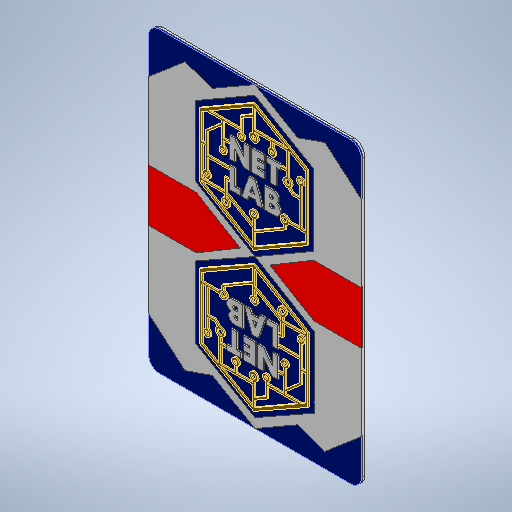
# Autodesk Inventor part: Aofwifi
Saved by Autodesk Inventor 2025 (Build 290162010, 162A)
## iProperties
Created: 2024-07-12
Part Number: Aofwifi
Material: Generic
Document SubType Name: Modeling
Designer: joshu
Density: 1 g/cm^3
Appearance: Default
Author: joshu
Autodesk Inventor part; units mm, degrees
(part 1 of 2)
ref_plane "YZ Plane" through (0, 0, 0) normal (1, 0, 0) x (0, 1, 0)
ref_plane "XZ Plane" through (0, 0, 0) normal (0, 1, 0) x (-1, 0, 0)
ref_plane "XY Plane" through (0, 0, 0) normal (0, 0, 1) x (1, 0, 0)
sketch "Sketch1" plane through (0, 0, 0) normal (0, 0, 1) x (1, 0, 0)
  line L0 (0, 0) -> (63.5, 0)
  line L1 (63.5, 0) -> (63.5, 88.9)
  line L2 (63.5, 88.9) -> (0, 88.9)
  line L3 (0, 88.9) -> (0, 0)
  line L4 (31.75, 44.45) -> (49.3079, 54.587)
  line L5 (49.3079, 54.587) -> (49.3079, 75.7826)
  line L6 (49.3079, 75.7826) -> (31.6801, 86.0828)
  line L7 (31.6801, 86.0828) -> (13.967, 75.8563)
  line L8 (13.967, 75.8563) -> (13.967, 55.04)
  line L9 (13.967, 55.04) -> (31.75, 44.45)
  line L10 (15.5263, 74.956) -> (31.6754, 84.2796)
  line L11 (31.6754, 84.2796) -> (47.7487, 74.8877)
  line L12 (47.7487, 74.8877) -> (47.7487, 55.4872)
  line L13 (47.7487, 55.4872) -> (31.7622, 46.2575)
  line L14 (31.7622, 46.2575) -> (15.5263, 55.9263)
  line L15 (15.5263, 55.9263) -> (15.5263, 74.956)
  line L16 (47.1273, 56.0392) -> (31.9379, 47.2671)
  line L17 (31.3664, 47.317) -> (16.2977, 56.192)
  line L18 (41.8086, 77.4972) -> (32.0418, 77.4972)
  line L19 (42.0908, 76.9257) -> (42.0908, 70.0939)
  line L20 (41.5193, 72.1376) -> (39.6994, 72.1376)
  line L21 (39.6994, 72.1376) -> (39.6994, 71.5661)
  line L22 (39.6994, 71.5661) -> (41.5193, 71.5661)
  arc A0 (31.465, 76.5861) -> (32.0365, 76.5861) centre (31.7507, 75.3324) ccw
  arc A1 (36.8763, 75.3571) -> (37.4478, 75.3571) centre (37.162, 74.2504) ccw
  circle A2 centre (37.162, 74.2504) radius 0.4762
  circle A3 centre (31.7507, 75.3324) radius 0.6191
  line L23 (45.9318, 69.8545) -> (45.9318, 58.9507)
  line L24 (45.3603, 66.7769) -> (43.3841, 66.7769)
  line L25 (43.1915, 66.2054) -> (45.3603, 66.2054)
  circle A4 centre (41.805, 68.7917) radius 0.762
  line L26 (43.1915, 66.2054) -> (41.9826, 67.4703)
  line L27 (43.3841, 66.7769) -> (42.5287, 67.6719)
  arc A5 (45.9318, 69.8545) -> (45.3603, 69.8545) centre (45.646, 70.9598) ccw
  circle A6 centre (45.646, 70.9598) radius 0.5715
  line L28 (40.6132, 56.5528) -> (40.6132, 57.4113)
  circle A7 centre (40.899, 58.665) radius 0.7144
  line L29 (32.0418, 83.1688) -> (32.0418, 77.4972)
  line L30 (32.0365, 76.9257) -> (32.0365, 76.5861)
  line L31 (32.0365, 76.9257) -> (36.8763, 76.9257)
  line L32 (36.8763, 75.3571) -> (36.8763, 76.9257)
  line L33 (37.4478, 76.9257) -> (37.4478, 75.3571)
  line L34 (37.4478, 76.9257) -> (41.5193, 76.9257)
  line L35 (42.0908, 76.9257) -> (42.7928, 76.9257)
  line L36 (32.0365, 83.1719) -> (41.8086, 77.4972)
  line L37 (42.7928, 76.9257) -> (47.1273, 74.4086)
  line L38 (41.5193, 70.0939) -> (41.5193, 71.5661)
  line L39 (41.5193, 72.1376) -> (41.5193, 76.9257)
  arc A8 (41.5193, 70.0939) -> (41.9826, 67.4703) centre (41.805, 68.7917) ccw
  arc A9 (42.5287, 67.6719) -> (42.0908, 70.0939) centre (41.805, 68.7917) ccw
  line L40 (45.3603, 58.9507) -> (45.3603, 66.2054)
  line L41 (45.3603, 66.7769) -> (45.3603, 69.8545)
  line L42 (47.1273, 58.9507) -> (45.9318, 58.9507)
  line L43 (45.3603, 58.9507) -> (42.1527, 58.9507)
  line L44 (42.1475, 58.3804) -> (47.1273, 58.3804)
  line L45 (41.1819, 57.4161) -> (41.1819, 56.2658)
  arc A10 (42.1527, 58.9507) -> (40.6132, 57.4113) centre (40.899, 58.665) ccw
  arc A11 (41.1819, 57.4161) -> (42.1475, 58.3804) centre (40.899, 58.665) ccw
  line L46 (47.1273, 74.4086) -> (47.1273, 58.9507)
  line L47 (47.1273, 58.3804) -> (47.1273, 56.0392)
  line L48 (27.6974, 78.6822) -> (27.6974, 79.0777)
  line L49 (28.2689, 78.6822) -> (31.465, 80.528)
  line L50 (27.6974, 79.0777) -> (31.465, 81.2535)
  line L51 (31.465, 76.5861) -> (31.465, 80.528)
  line L52 (31.465, 81.2535) -> (31.465, 83.1596)
  line L53 (31.9379, 51.4601) -> (40.6132, 56.5528)
  line L54 (31.9379, 50.8392) -> (41.1819, 56.2658)
  line L55 (16.2977, 57.1448) -> (22.9994, 57.1448)
  line L56 (22.9994, 56.5733) -> (16.2977, 56.5733)
  line L57 (16.2977, 56.5733) -> (16.2977, 57.1448)
  line L58 (22.9994, 60.9472) -> (23.5709, 60.9472)
  line L59 (22.9994, 60.9472) -> (24.4329, 60.9472)
  line L60 (24.4329, 60.9472) -> (24.4329, 60.3757)
  line L61 (24.4329, 60.3757) -> (23.5709, 60.3757)
  line L62 (22.9994, 60.3757) -> (22.9994, 60.9472)
  line L63 (23.5709, 56.4373) -> (31.3664, 51.9861)
  line L64 (31.3664, 52.5972) -> (23.5709, 57.0484)
  arc A12 (31.9379, 54.3552) -> (31.3664, 54.3552) centre (31.6521, 55.5111) ccw
  circle A13 centre (31.6521, 55.5111) radius 0.6191
  arc A14 (22.9994, 55.5805) -> (23.5709, 55.5805) centre (23.2852, 54.3309) ccw
  circle A15 centre (23.2852, 54.3309) radius 0.7144
  line L65 (23.5709, 60.3757) -> (23.5709, 57.0484)
  line L66 (23.5709, 56.4373) -> (23.5709, 55.5805)
  line L67 (22.9994, 55.5805) -> (22.9994, 56.5733)
  line L68 (22.9994, 57.1448) -> (22.9994, 60.9472)
  line L69 (31.3664, 54.3552) -> (31.3664, 52.5972)
  line L70 (31.3664, 51.9861) -> (31.3664, 47.317)
  line L71 (31.9379, 47.2671) -> (31.9379, 50.8392)
  line L72 (31.9379, 51.4601) -> (31.9379, 54.3552)
  arc A16 (27.6974, 74.6924) -> (28.2689, 74.6924) centre (27.9831, 73.6844) ccw
  circle A17 centre (27.9831, 73.6844) radius 0.4763
  line L73 (18.5492, 75.7007) -> (27.6974, 75.7007)
  line L74 (22.769, 70.6818) -> (24.4329, 70.6818)
  line L75 (24.4329, 70.6818) -> (24.4329, 70.1103)
  line L76 (24.4329, 70.1103) -> (22.769, 70.1103)
  line L77 (22.769, 70.1103) -> (22.769, 70.2009)
  line L78 (16.2977, 66.7769) -> (17.4065, 66.7769)
  line L79 (17.978, 66.7769) -> (17.978, 66.2054)
  line L80 (17.4065, 66.2054) -> (16.2977, 66.2054)
  line L81 (17.978, 63.9706) -> (24.4329, 63.9706)
  line L82 (24.4329, 63.9706) -> (24.4329, 63.3991)
  line L83 (24.4329, 63.3991) -> (17.978, 63.3991)
  line L84 (17.4065, 66.7769) -> (17.4065, 70.2549)
  line L85 (17.978, 70.0307) -> (17.978, 66.7769)
  line L86 (17.4065, 70.2549) -> (22.1975, 74.4365)
  line L87 (17.978, 70.0307) -> (22.1975, 73.7135)
  arc A18 (22.1975, 68.5281) -> (22.769, 68.5281) centre (22.4833, 67.4703) ccw
  circle A19 centre (22.4833, 67.4703) radius 0.5239
  line L88 (16.2977, 74.4004) -> (17.5596, 75.1292)
  line L89 (18.5492, 75.7007) -> (31.465, 83.1596)
  line L90 (27.6974, 75.1292) -> (22.769, 75.1292)
  line L91 (22.1975, 75.1292) -> (17.5596, 75.1292)
  line L92 (22.1975, 74.4365) -> (22.1975, 75.1292)
  line L93 (28.2689, 74.6924) -> (28.2689, 78.6822)
  line L94 (22.769, 75.1292) -> (22.769, 70.6818)
  line L95 (22.769, 70.1103) -> (22.769, 68.5281)
  line L96 (22.1975, 67.8875) -> (22.1975, 67.9094)
  line L97 (22.1975, 68.5281) -> (22.1975, 73.7135)
  line L98 (16.2977, 56.192) -> (16.2977, 66.2054)
  line L99 (16.2977, 66.7769) -> (16.2977, 74.4004)
  line L100 (17.978, 63.9706) -> (17.978, 66.2054)
  line L101 (27.6974, 78.6822) -> (27.6974, 75.7007)
  line L102 (27.6974, 75.1292) -> (27.6974, 74.6924)
  line L103 (24.4329, 66.1976) -> (26.1474, 66.1976)
  line L104 (26.1474, 66.1976) -> (26.1474, 69.7075)
  line L105 (26.1474, 72.4542) -> (24.4329, 72.4542)
  line L106 (24.4329, 72.4542) -> (24.4329, 66.1976)
  line L107 (28.7777, 72.4542) -> (30.4922, 72.4542)
  line L108 (30.4922, 72.4542) -> (30.4922, 66.1976)
  line L109 (30.4922, 66.1976) -> (28.7777, 66.1976)
  line L110 (28.7777, 68.9443) -> (28.7777, 72.4542)
  line L111 (28.7777, 66.1976) -> (26.1474, 69.7075)
  line L112 (26.1474, 72.4542) -> (28.7777, 68.9443)
  line L113 (31.2537, 72.4542) -> (32.9682, 72.4542)
  line L114 (32.9682, 66.1976) -> (31.2537, 66.1976)
  line L115 (31.2537, 66.1976) -> (31.2537, 72.4542)
  line L116 (31.2537, 72.4542) -> (34.8385, 72.4542)
  line L117 (34.8385, 72.4542) -> (34.8385, 70.7397)
  line L118 (34.8385, 70.7397) -> (32.9682, 70.7397)
  line L119 (31.2537, 70.7397) -> (31.2537, 72.4542)
  line L120 (32.9682, 70.0633) -> (34.8385, 70.0633)
  line L121 (34.8385, 70.0633) -> (34.8385, 68.5393)
  line L122 (34.8385, 68.5393) -> (32.9682, 68.5393)
  line L123 (31.2537, 68.5393) -> (31.2537, 70.0633)
  line L124 (31.2537, 66.1976) -> (34.8385, 66.1976)
  line L125 (34.8385, 66.1976) -> (34.8385, 67.9121)
  line L126 (34.8385, 67.9121) -> (32.9682, 67.9121)
  line L127 (31.2537, 67.9121) -> (31.2537, 66.1976)
  line L128 (32.9682, 70.7397) -> (32.9682, 70.0633)
  line L129 (32.9682, 68.5393) -> (32.9682, 67.9121)
  line L130 (39.6994, 72.4422) -> (35.4849, 72.4422)
  line L131 (35.4849, 72.4422) -> (35.4849, 70.9182)
  line L132 (39.6994, 70.9182) -> (39.6994, 72.4422)
  line L133 (38.4466, 70.9182) -> (38.4466, 66.1976)
  line L134 (38.4466, 66.1976) -> (36.7321, 66.1976)
  line L135 (36.7321, 66.1976) -> (36.7321, 70.9182)
  line L136 (36.7321, 70.9182) -> (36.8763, 70.9182)
  line L137 (35.4849, 70.9182) -> (36.7321, 70.9182)
  line L138 (38.4466, 70.9182) -> (39.6994, 70.9182)
  line L139 (24.4329, 64.6461) -> (26.1474, 64.6461)
  line L140 (26.1474, 64.6461) -> (26.1474, 59.9044)
  line L141 (26.1474, 58.3804) -> (24.4329, 58.3804)
  line L142 (24.4329, 58.3804) -> (24.4329, 64.6461)
  line L143 (24.4329, 58.3804) -> (27.8234, 58.3804)
  line L144 (27.8234, 58.3804) -> (27.8234, 59.9044)
  line L145 (27.8234, 59.9044) -> (26.1474, 59.9044)
  line L146 (24.4329, 59.9044) -> (24.4329, 58.3804)
  line L147 (28.1466, 58.3804) -> (29.8611, 58.3804)
  line L148 (29.8611, 58.3804) -> (30.3254, 59.5144)
  line L149 (30.3254, 59.5144) -> (32.2304, 59.5144)
  line L150 (30.3254, 64.6461) -> (32.2304, 64.6461)
  line L151 (28.1466, 58.3804) -> (30.3254, 64.6461)
  line L152 (32.728, 58.3804) -> (34.4425, 58.3804)
  line L153 (32.728, 58.3804) -> (32.2304, 59.5144)
  line L154 (34.4425, 58.3804) -> (32.2304, 64.6461)
  line L155 (30.6203, 60.8236) -> (31.9379, 60.8236)
  line L156 (31.9379, 60.8236) -> (31.2779, 62.4085)
  line L157 (31.2779, 62.4085) -> (30.6203, 60.8236)
  line L158 (34.9216, 58.3804) -> (34.9216, 64.6461)
  line L159 (34.9216, 64.6461) -> (37.8691, 64.6461)
  line L160 (34.9216, 58.3804) -> (37.8691, 58.3804)
  line L161 (36.5599, 59.8143) -> (36.5599, 60.939)
  line L162 (36.5599, 62.1736) -> (36.5599, 63.1944)
  line L163 (36.5599, 63.1944) -> (37.2133, 63.1944)
  line L164 (36.5599, 62.1736) -> (37.2133, 62.1736)
  arc A20 (37.2133, 62.1736) -> (37.2133, 63.1944) centre (37.055, 62.684) ccw
  line L165 (36.5599, 60.939) -> (37.4519, 60.939)
  line L166 (36.5599, 59.8143) -> (37.4396, 59.8143)
  arc A21 (37.4396, 59.8143) -> (37.4519, 60.939) centre (37.3959, 60.3772) ccw
  arc A22 (38.5631, 61.7817) -> (37.8691, 64.6461) centre (37.5266, 63.0469) ccw
  arc A23 (37.8691, 58.3804) -> (38.5631, 61.7817) centre (37.9604, 60.1332) ccw
  arc A24 (17.4065, 59.8724) -> (17.978, 59.8724) centre (17.6923, 58.815) ccw
  circle A25 centre (17.6923, 58.815) radius 0.5239
  line L167 (17.4065, 66.2054) -> (17.4065, 59.8724)
  line L168 (17.978, 59.8724) -> (17.978, 63.3991)
  line L169 (32.0418, 83.1688) -> (41.8086, 77.4972)
  line L170 (32.0418, 77.4972) -> (41.8086, 77.4972)
  line L171 (32.0418, 77.4972) -> (32.0418, 83.1688)
  line L172 (0, 44.45) -> (63.5, 44.45) construction
  line L173 (31.75, 88.9) -> (31.75, 0) construction
  line L174 (0, 52.2573) -> (14.2102, 52.2573)
  line L175 (14.2102, 52.2573) -> (27.3204, 44.45)
  line L176 (0, 36.6427) -> (14.2102, 36.6427)
  line L177 (14.2102, 36.6427) -> (27.3204, 44.45)
  line L178 (63.5, 52.2573) -> (49.2898, 52.2573)
  line L179 (49.2898, 52.2573) -> (36.1796, 44.45)
  line L180 (49.2898, 36.6427) -> (36.1796, 44.45)
  line L181 (63.5, 36.6427) -> (49.2898, 36.6427)
  line L182 (0, 75.0796) -> (10.8905, 84.3747)
  line L183 (10.8905, 84.3747) -> (18.9583, 81.5148)
  line L184 (18.9583, 81.5148) -> (31.75, 88.9)
  line L185 (63.5, 75.0796) -> (52.6095, 84.3747)
  line L186 (52.6095, 84.3747) -> (44.5417, 81.5148)
  line L187 (44.5417, 81.5148) -> (31.75, 88.9)
  line L188 (46.0393, 22.6946) -> (47.1481, 22.6946)
  line L189 (45.4678, 22.1231) -> (45.4678, 22.6946)
  line L190 (45.4678, 24.9294) -> (45.4678, 22.6946)
  line L191 (47.1481, 22.1231) -> (46.0393, 22.1231)
  line L192 (47.1481, 32.3267) -> (47.1481, 31.7552)
  line L193 (47.1481, 32.708) -> (47.1481, 22.6946)
  line L194 (47.1481, 31.7552) -> (40.4464, 31.7552)
  line L195 (40.4464, 32.3267) -> (47.1481, 32.3267)
  line L196 (45.4678, 29.0276) -> (45.4678, 25.5009)
  line L197 (46.0393, 22.6946) -> (46.0393, 29.0276)
  circle A26 centre (45.7535, 30.085) radius 0.5239
  arc A27 (46.0393, 29.0276) -> (45.4678, 29.0276) centre (45.7535, 30.085) ccw
  line L198 (20.6531, 11.9743) -> (16.3185, 14.4914)
  line L199 (21.355, 11.9743) -> (20.6531, 11.9743)
  line L200 (21.9265, 16.7624) -> (21.9265, 11.9743)
  line L201 (21.355, 11.9743) -> (21.355, 18.8061)
  line L202 (21.9265, 16.7624) -> (23.7464, 16.7624)
  line L203 (23.7464, 17.3339) -> (21.9265, 17.3339)
  line L204 (25.998, 11.9743) -> (21.9265, 11.9743)
  line L205 (26.5695, 13.5429) -> (26.5695, 11.9743)
  circle A28 centre (21.6408, 20.1083) radius 0.762
  circle A29 centre (26.2838, 14.6496) radius 0.4762
  arc A30 (26.5695, 13.5429) -> (25.998, 13.5429) centre (26.2838, 14.6496) ccw
  line L206 (31.4093, 11.9743) -> (26.5695, 11.9743)
  arc A31 (31.9808, 12.3139) -> (31.4093, 12.3139) centre (31.6951, 13.5676) ccw
  line L207 (25.998, 11.9743) -> (25.998, 13.5429)
  line L208 (45.4678, 24.9294) -> (39.013, 24.9294)
  line L209 (39.013, 25.5009) -> (45.4678, 25.5009)
  line L210 (39.013, 24.9294) -> (39.013, 25.5009)
  circle A32 centre (40.1606, 34.5691) radius 0.7144
  arc A33 (40.4464, 33.3195) -> (39.8749, 33.3195) centre (40.1606, 34.5691) ccw
  line L211 (39.8749, 32.4627) -> (39.8749, 33.3195)
  line L212 (40.4464, 33.3195) -> (40.4464, 32.3267)
  line L213 (39.013, 27.9528) -> (39.013, 28.5243)
  line L214 (39.8749, 28.5243) -> (39.8749, 31.8516)
  line L215 (39.013, 28.5243) -> (39.8749, 28.5243)
  line L216 (40.4464, 31.7552) -> (40.4464, 27.9528)
  line L217 (40.4464, 28.5243) -> (40.4464, 27.9528)
  line L218 (40.4464, 27.9528) -> (39.8749, 27.9528)
  line L219 (40.4464, 27.9528) -> (39.013, 27.9528)
  line L220 (33.5847, 30.5196) -> (33.1204, 29.3856)
  line L221 (35.6224, 28.9956) -> (37.2985, 28.9956)
  line L222 (35.2992, 30.5196) -> (33.5847, 30.5196)
  line L223 (39.013, 28.9956) -> (39.013, 30.5196)
  line L224 (35.2992, 30.5196) -> (33.1204, 24.2539)
  line L225 (46.0393, 18.6451) -> (41.2483, 14.4635)
  line L226 (45.4678, 18.8693) -> (41.2483, 15.1865)
  line L227 (40.6768, 18.7897) -> (40.6768, 20.3719)
  line L228 (41.2483, 21.0125) -> (41.2483, 20.9906)
  line L229 (41.2483, 20.3719) -> (41.2483, 15.1865)
  line L230 (40.6768, 13.7708) -> (40.6768, 18.2182)
  line L231 (41.2483, 14.4635) -> (41.2483, 13.7708)
  line L232 (41.2483, 13.7708) -> (45.8862, 13.7708)
  line L233 (47.1481, 22.1231) -> (47.1481, 14.4996)
  line L234 (47.1481, 14.4996) -> (45.8862, 13.7708)
  circle A34 centre (40.9626, 21.4297) radius 0.5239
  line L235 (32.8255, 28.0764) -> (31.5079, 28.0764)
  line L236 (32.1679, 26.4915) -> (32.8255, 28.0764)
  line L237 (31.5079, 28.0764) -> (32.1679, 26.4915)
  line L238 (33.1204, 29.3856) -> (31.2154, 29.3856)
  line L239 (35.6224, 30.5196) -> (35.6224, 28.9956)
  line L240 (37.2985, 24.2539) -> (37.2985, 28.9956)
  line L241 (37.2985, 30.5196) -> (39.013, 30.5196)
  line L242 (39.013, 30.5196) -> (39.013, 24.2539)
  line L243 (39.013, 30.5196) -> (35.6224, 30.5196)
  line L244 (39.013, 24.2539) -> (37.2985, 24.2539)
  line L245 (33.1204, 24.2539) -> (31.2154, 24.2539)
  line L246 (30.7178, 30.5196) -> (31.2154, 29.3856)
  line L247 (37.2985, 16.4458) -> (39.013, 16.4458)
  line L248 (40.6768, 18.2182) -> (39.013, 18.2182)
  line L249 (39.013, 18.7897) -> (40.6768, 18.7897)
  line L250 (40.6768, 18.7897) -> (40.6768, 18.6991)
  line L251 (39.013, 18.2182) -> (39.013, 18.7897)
  line L252 (46.0393, 22.1231) -> (46.0393, 18.6451)
  line L253 (45.4678, 18.8693) -> (45.4678, 22.1231)
  arc A35 (41.2483, 20.3719) -> (40.6768, 20.3719) centre (40.9626, 21.4297) ccw
  line L254 (39.013, 16.4458) -> (39.013, 22.7024)
  line L255 (39.013, 22.7024) -> (37.2985, 22.7024)
  line L256 (32.9536, 22.7024) -> (34.6681, 22.7024)
  line L257 (30.4777, 22.7024) -> (32.1922, 22.7024)
  line L258 (30.4777, 18.8367) -> (28.6073, 18.8367)
  line L259 (32.1922, 22.7024) -> (28.6073, 22.7024)
  line L260 (28.6073, 22.7024) -> (28.6073, 20.9879)
  line L261 (28.6073, 20.9879) -> (30.4777, 20.9879)
  line L262 (32.1922, 20.9879) -> (32.1922, 22.7024)
  line L263 (30.4777, 20.3607) -> (30.4777, 20.9879)
  line L264 (28.6073, 20.3607) -> (30.4777, 20.3607)
  line L265 (28.6073, 18.8367) -> (28.6073, 20.3607)
  line L266 (32.1922, 20.3607) -> (32.1922, 18.8367)
  line L267 (30.4777, 18.1603) -> (30.4777, 18.8367)
  line L268 (26.8859, 25.7056) -> (26.2325, 25.7056)
  line L269 (26.8859, 29.0857) -> (26.0062, 29.0857)
  line L270 (26.8859, 27.961) -> (25.9939, 27.961)
  line L271 (28.5242, 30.5196) -> (25.5767, 30.5196)
  line L272 (32.0794, 36.9139) -> (32.0794, 41.583)
  line L273 (31.5079, 41.6329) -> (31.5079, 38.0608)
  line L274 (26.8859, 26.7264) -> (26.8859, 25.7056)
  line L275 (28.5242, 24.2539) -> (25.5767, 24.2539)
  line L276 (29.0033, 30.5196) -> (31.2154, 24.2539)
  line L277 (30.7178, 30.5196) -> (29.0033, 30.5196)
  line L278 (26.8859, 26.7264) -> (26.2325, 26.7264)
  line L279 (28.5242, 30.5196) -> (28.5242, 24.2539)
  arc A36 (26.2325, 26.7264) -> (26.2325, 25.7056) centre (26.3908, 26.216) ccw
  line L280 (26.8859, 29.0857) -> (26.8859, 27.961)
  arc A37 (26.0062, 29.0857) -> (25.9939, 27.961) centre (26.0499, 28.5228) ccw
  arc A38 (24.8827, 27.1183) -> (25.5767, 24.2539) centre (25.9192, 25.8531) ccw
  arc A39 (25.5767, 30.5196) -> (24.8827, 27.1183) centre (25.4854, 28.7668) ccw
  line L281 (23.7464, 16.7624) -> (23.7464, 17.3339)
  line L282 (24.9992, 22.7024) -> (26.7137, 22.7024)
  line L283 (27.961, 17.9818) -> (26.7137, 17.9818)
  line L284 (26.7137, 22.7024) -> (26.7137, 17.9818)
  line L285 (26.7137, 17.9818) -> (26.5695, 17.9818)
  line L286 (24.9992, 17.9818) -> (24.9992, 22.7024)
  line L287 (24.9992, 17.9818) -> (23.7464, 17.9818)
  line L288 (27.961, 16.4578) -> (27.961, 17.9818)
  line L289 (23.7464, 16.4578) -> (27.961, 16.4578)
  line L290 (23.7464, 17.9818) -> (23.7464, 16.4578)
  line L291 (31.75, 44.45) -> (14.1379, 34.5158)
  line L292 (15.6972, 33.6051) -> (31.7276, 42.6471)
  line L293 (16.3185, 32.8608) -> (31.5079, 41.6329)
  line L294 (31.5079, 37.4399) -> (22.8326, 32.3472)
  line L295 (31.5079, 38.0608) -> (22.2639, 32.6342)
  line L296 (31.5079, 37.4399) -> (31.5079, 34.5448)
  line L297 (35.7484, 10.2178) -> (35.7484, 9.8223)
  line L298 (35.1769, 10.2178) -> (31.9808, 8.372)
  line L299 (35.7484, 9.8223) -> (31.9808, 7.6465)
  line L300 (31.9808, 12.3139) -> (31.9808, 8.372)
  line L301 (31.9808, 7.6465) -> (31.9808, 5.7404)
  circle A40 centre (35.4627, 15.2156) radius 0.4763
  arc A41 (35.7484, 14.2076) -> (35.1769, 14.2076) centre (35.4627, 15.2156) ccw
  line L302 (35.7484, 13.7708) -> (35.7484, 14.2076)
  line L303 (35.7484, 13.7708) -> (40.6768, 13.7708)
  line L304 (44.8966, 13.1993) -> (35.7484, 13.1993)
  line L305 (35.1769, 14.2076) -> (35.1769, 10.2178)
  line L306 (35.7484, 10.2178) -> (35.7484, 13.1993)
  line L307 (44.8966, 13.1993) -> (31.9808, 5.7404)
  line L308 (31.4093, 11.9743) -> (31.4093, 12.3139)
  line L309 (47.9195, 13.7706) -> (31.7623, 4.657)
  circle A42 centre (31.6951, 13.5676) radius 0.6191
  line L310 (31.7499, 2.8598) -> (49.4788, 12.8599)
  line L311 (47.9195, 32.9751) -> (47.9195, 13.7706)
  line L312 (49.4788, 12.8599) -> (49.4788, 33.86)
  circle A43 centre (31.7937, 33.3889) radius 0.6191
  line L313 (32.0794, 41.583) -> (47.1481, 32.708)
  line L314 (49.4788, 33.86) -> (31.75, 44.45)
  line L315 (31.7276, 42.6471) -> (47.9195, 32.9751)
  line L316 (32.0794, 36.3028) -> (39.8749, 31.8516)
  line L317 (39.8749, 32.4627) -> (32.0794, 36.9139)
  line L318 (32.0794, 34.5448) -> (32.0794, 36.3028)
  arc A44 (31.5079, 34.5448) -> (32.0794, 34.5448) centre (31.7937, 33.3889) ccw
  circle A45 centre (17.7998, 17.9402) radius 0.5715
  line L319 (18.0855, 22.1231) -> (20.0617, 22.1231)
  line L320 (20.2543, 22.6946) -> (18.0855, 22.6946)
  line L321 (22.8326, 32.3472) -> (22.8326, 31.4887)
  circle A46 centre (22.5468, 30.235) radius 0.7144
  line L322 (21.2984, 30.5196) -> (16.3185, 30.5196)
  line L323 (22.2639, 31.4839) -> (22.2639, 32.6342)
  arc A47 (21.2931, 29.9493) -> (22.8326, 31.4887) centre (22.5468, 30.235) ccw
  arc A48 (22.2639, 31.4839) -> (21.2984, 30.5196) centre (22.5468, 30.235) ccw
  line L324 (16.3185, 30.5196) -> (16.3185, 32.8608)
  line L325 (14.1379, 34.5158) -> (14.1379, 13.1174)
  line L326 (15.6972, 14.0137) -> (15.6972, 33.6051)
  line L327 (17.514, 19.0455) -> (17.514, 29.9493)
  line L328 (20.2543, 22.6946) -> (21.4633, 21.4297)
  line L329 (20.0617, 22.1231) -> (20.9171, 21.2281)
  arc A49 (17.514, 19.0455) -> (18.0855, 19.0455) centre (17.7998, 17.9402) ccw
  line L330 (21.9265, 18.8061) -> (21.9265, 17.3339)
  arc A50 (20.9171, 21.2281) -> (21.355, 18.8061) centre (21.6408, 20.1083) ccw
  line L331 (18.0855, 22.1231) -> (18.0855, 19.0455)
  line L332 (16.3185, 14.4914) -> (16.3185, 29.9493)
  line L333 (16.3185, 29.9493) -> (17.514, 29.9493)
  line L334 (18.0855, 29.9493) -> (18.0855, 22.6946)
  line L335 (18.0855, 29.9493) -> (21.2931, 29.9493)
  arc A51 (21.9265, 18.8061) -> (21.4633, 21.4297) centre (21.6408, 20.1083) ccw
  line L336 (14.1379, 13.1174) -> (31.7499, 2.8598)
  line L337 (31.7623, 4.657) -> (15.6972, 14.0137)
  line L338 (21.6372, 11.4028) -> (31.404, 11.4028)
  line L339 (31.404, 11.4028) -> (31.404, 5.7312)
  line L340 (31.404, 5.7312) -> (21.6372, 11.4028)
  line L341 (37.2985, 22.7024) -> (37.2985, 19.1925)
  line L342 (34.6681, 16.4458) -> (32.9536, 16.4458)
  line L343 (32.9536, 16.4458) -> (32.9536, 22.7024)
  line L344 (34.6681, 22.7024) -> (37.2985, 19.1925)
  line L345 (28.6073, 18.1603) -> (30.4777, 18.1603)
  line L346 (32.1922, 16.4458) -> (28.6073, 16.4458)
  line L347 (28.6073, 16.4458) -> (28.6073, 18.1603)
  line L348 (32.1922, 22.7024) -> (32.1922, 16.4458)
  line L349 (32.1922, 16.4458) -> (30.4777, 16.4458)
  line L350 (34.6681, 19.9557) -> (34.6681, 16.4458)
  line L351 (37.2985, 16.4458) -> (34.6681, 19.9557)
  line L352 (32.1922, 18.1603) -> (32.1922, 16.4458)
  line L353 (0, 13.8204) -> (10.8905, 4.5253)
  line L354 (10.8905, 4.5253) -> (18.9583, 7.3852)
  line L355 (18.9583, 7.3852) -> (31.75, 0)
  line L356 (63.5, 13.8204) -> (52.6095, 4.5253)
  line L357 (52.6095, 4.5253) -> (44.5417, 7.3852)
  line L358 (44.5417, 7.3852) -> (31.75, 0)
  point P0 (31.9379, 47.317)
  point P1 (31.7229, 65.2666)
  point P2 (31.7229, 23.6334)
  point P3 (31.7229, 23.6334)
  point P4 (31.9379, 5.6837)
  point P5 (63.5, 75.0796)
  dimension "d0" = 63.5
  dimension "d1" = 88.9
  dimension "d43" = 44.45
  dimension "d99" = 120
  constraints: 718 end point, 170 parallel, 64 point on circle, 50 centre point, 42 perpendicular, 36 horizontal, 21 point on line, 20 coincident, 19 symmetric about line, 7 collinear, 5 midpoint, 4 vertical, 17 other
  measures "d0" distance of L2.end L1.end
  measures "d1" distance of L1.end L0.end
  measures "d43" distance between parallel lines of L172 L2
  measures "d99" angle of L357 L356
extrude "Extrusion1" add sketch "Sketch1" along normal blind 0.4 contours L3 L353 L354 L355 L0 | L358 L357 L356 L1 L0 | L3 L2 L184 L183 L182 | L185 L186 L187 L2 L1 | L9 L8 L7 L6 L5 L4 | L314 L312 L310 L336 L325 L291 | L10 L11 L12 L13 L14 L15 | L16 L71 L54 L45 A11 L44 L47 | L17 L98 L56 L67 A14 L66 L63 L70 | L18 L29 L36 | L35 L37 L46 L42 L23 A5 L41 L24 L27 A9 L19 | L20 L132 L130 L131 L137 L135 L134 L133 L138 L22 L38 A8 L26 L25 L40 L43 A10 L28 L53 L72 A12 L69 L64 L65 L61 L142 L141 L143 L144 L145 L140 L139 L81 L100 L79 L85 L87 L97 A18 L95 L76 L106 L103 L104 L111 L109 L108 L107 L110 L112 L105 L74 L94 L90 L102 A16 L93 L49 L51 A0 L30 L31 L32 A1 L33 L34 L39 | L21 L132 L138 L133 L134 L135 L137 L131 L130 | L106 L105 L112 L110 L107 L108 L109 L111 L104 L103 L75 | L60 L142 L82 L139 L140 L145 L144 L143 L141 | L59 L58 L62 L68 L55 L98 L80 L167 A24 L168 L83 L142 | A2 | A3 | A4 | A6 | A7 | L101 L73 L89 L52 L50 L48 | A13 | A15 | A17 | L99 L88 L91 L92 L86 L84 L78 | A19 | L113 L116 L117 L118 L128 L120 L121 L122 L129 L126 L125 L124 L114 L115 | L151 L150 L154 L152 L153 L149 L148 L147 | L157 L156 L155 | L158 L159 A22 A23 L160 | L161 L165 A21 L166 | L162 L163 A20 L164 | A25 | L197 A27 L196 L209 L242 L219 L218 L216 L194 L193 L188 | L210 L242 L244 L240 L221 L239 L243 L241 L223 L213 | L208 L190 L189 L253 L226 L229 A35 L227 L249 L254 L255 L341 L344 L256 L343 L342 L350 L351 L247 L248 L230 L303 L302 A41 L305 L298 L300 A31 L308 L206 L205 A30 L207 L204 L200 L202 L290 L289 L288 L283 L284 L282 L286 L287 L203 L330 A51 L328 L320 L334 L335 A47 L321 L294 L296 A44 L318 L316 L214 L215 L242 L223 L241 L243 L239 L221 L240 L244 | L251 L254 L247 L351 L350 L342 L343 L256 L344 L341 L255 | L290 L287 L286 L282 L284 L283 L288 L289 L281 | L233 L234 L232 L231 L225 L252 L191 | L193 L195 L212 A33 L211 L317 L272 L313 | A26 | L198 L332 L333 L327 A49 L331 L319 L329 A50 L201 L199 | A28 | A29 | A32 | L222 L224 L245 L276 L277 L246 L238 L220 | A34 | L236 L237 L235 | L257 L262 L348 L266 L346 L347 L345 L267 L258 L265 L264 L263 L261 L260 L259 | L268 A36 L278 L274 | L280 L270 A37 L269 | L279 L275 A38 A39 L271 | L273 L295 L323 A48 L322 L324 L293 | L292 L315 L311 L309 L337 L326 | L306 L304 L307 L301 L299 L297 | A40 | A42 | A43 | A45 | A46 | L338 L339 L340
extrude "Extrusion12" add sketch "Sketch1" along normal blind 0.4 separate body contours L3 L174 L175 L177 L176 | L181 L180 L179 L178 L1
extrude "Extrusion13" add sketch "Sketch1" along normal blind 0.4 separate body contours L355 L354 L353 L3 L176 L177 L175 L174 L182 L183 L184 L187 L186 L185 L1 L178 L179 L180 L181 L356 L357 L358
extrude "Extrusion14" add sketch "Sketch1" against normal blind 0.4 contours L21 L132 L138 L133 L134 L135 L137 L131 L130 | L106 L105 L112 L110 L107 L108 L109 L111 L104 L103 L75 | L60 L142 L82 L139 L140 L145 L144 L143 L141 | L113 L116 L117 L118 L128 L120 L121 L122 L129 L126 L125 L124 L114 L115 | L151 L150 L154 L152 L153 L149 L148 L147 | L158 L159 A22 A23 L160 | L210 L242 L244 L240 L221 L239 L243 L241 L223 L213 | L251 L254 L247 L351 L350 L342 L343 L256 L344 L341 L255 | L290 L287 L286 L282 L284 L283 L288 L289 L281 | L222 L224 L245 L276 L277 L246 L238 L220 | L257 L262 L348 L266 L346 L347 L345 L267 L258 L265 L264 L263 L261 L260 L259 | L279 L275 A38 A39 L271 bodies 3
extrude "Extrusion15" add sketch "Sketch1" against normal blind 0.4 separate body contours L10 L11 L12 L13 L14 L15 | L292 L315 L311 L309 L337 L326
pattern_linear "Rectangular Pattern1" count 2 spacing 0.8 along (0, 0, 1) of "Extrusion15" bodies 4
pattern_linear "Rectangular Pattern2" count 2 spacing 0.8 along (0, 0, 1) of "Extrusion14" bodies 3
extrude "Extrusion16" cut sketch "Sketch1" against normal blind 0.4 contours L9 L8 L7 L6 L5 L4 | L314 L312 L310 L336 L325 L291 | L10 L11 L12 L13 L14 L15 | L16 L71 L54 L45 A11 L44 L47 | L17 L98 L56 L67 A14 L66 L63 L70 | L18 L29 L36 | L35 L37 L46 L42 L23 A5 L41 L24 L27 A9 L19 | L20 L132 L130 L131 L137 L135 L134 L133 L138 L22 L38 A8 L26 L25 L40 L43 A10 L28 L53 L72 A12 L69 L64 L65 L61 L142 L141 L143 L144 L145 L140 L139 L81 L100 L79 L85 L87 L97 A18 L95 L76 L106 L103 L104 L111 L109 L108 L107 L110 L112 L105 L74 L94 L90 L102 A16 L93 L49 L51 A0 L30 L31 L32 A1 L33 L34 L39 | L21 L132 L138 L133 L134 L135 L137 L131 L130 | L106 L105 L112 L110 L107 L108 L109 L111 L104 L103 L75 | L60 L142 L82 L139 L140 L145 L144 L143 L141 | L59 L58 L62 L68 L55 L98 L80 L167 A24 L168 L83 L142 | A2 | A3 | A4 | A6 | A7 | L101 L73 L89 L52 L50 L48 | A13 | A15 | A17 | L99 L88 L91 L92 L86 L84 L78 | A19 | L113 L116 L117 L118 L128 L120 L121 L122 L129 L126 L125 L124 L114 L115 | L151 L150 L154 L152 L153 L149 L148 L147 | L157 L156 L155 | L158 L159 A22 A23 L160 | L161 L165 A21 L166 | L162 L163 A20 L164 | A25 | L197 A27 L196 L209 L242 L219 L218 L216 L194 L193 L188 | L210 L242 L244 L240 L221 L239 L243 L241 L223 L213 | L208 L190 L189 L253 L226 L229 A35 L227 L249 L254 L255 L341 L344 L256 L343 L342 L350 L351 L247 L248 L230 L303 L302 A41 L305 L298 L300 A31 L308 L206 L205 A30 L207 L204 L200 L202 L290 L289 L288 L283 L284 L282 L286 L287 L203 L330 A51 L328 L320 L334 L335 A47 L321 L294 L296 A44 L318 L316 L214 L215 L242 L223 L241 L243 L239 L221 L240 L244 | L251 L254 L247 L351 L350 L342 L343 L256 L344 L341 L255 | L290 L287 L286 L282 L284 L283 L288 L289 L281 | L233 L234 L232 L231 L225 L252 L191 | L193 L195 L212 A33 L211 L317 L272 L313 | A26 | L198 L332 L333 L327 A49 L331 L319 L329 A50 L201 L199 | A28 | A29 | A32 | L222 L224 L245 L276 L277 L246 L238 L220 | A34 | L236 L237 L235 | L257 L262 L348 L266 L346 L347 L345 L267 L258 L265 L264 L263 L261 L260 L259 | L268 A36 L278 L274 | L280 L270 A37 L269 | L279 L275 A38 A39 L271 | L273 L295 L323 A48 L322 L324 L293 | L292 L315 L311 L309 L337 L326 | L306 L304 L307 L301 L299 L297 | A40 | A42 | A43 | A45 | A46 | L338 L339 L340 bodies 3
extrude "Extrusion17" cut sketch "Sketch1" against normal blind 25.4 contours L9 L8 L7 L6 L5 L4 | L314 L312 L310 L336 L325 L291 | L10 L11 L12 L13 L14 L15 | L16 L71 L54 L45 A11 L44 L47 | L17 L98 L56 L67 A14 L66 L63 L70 | L18 L29 L36 | L35 L37 L46 L42 L23 A5 L41 L24 L27 A9 L19 | L20 L132 L130 L131 L137 L135 L134 L133 L138 L22 L38 A8 L26 L25 L40 L43 A10 L28 L53 L72 A12 L69 L64 L65 L61 L142 L141 L143 L144 L145 L140 L139 L81 L100 L79 L85 L87 L97 A18 L95 L76 L106 L103 L104 L111 L109 L108 L107 L110 L112 L105 L74 L94 L90 L102 A16 L93 L49 L51 A0 L30 L31 L32 A1 L33 L34 L39 | L21 L132 L138 L133 L134 L135 L137 L131 L130 | L106 L105 L112 L110 L107 L108 L109 L111 L104 L103 L75 | L60 L142 L82 L139 L140 L145 L144 L143 L141 | L59 L58 L62 L68 L55 L98 L80 L167 A24 L168 L83 L142 | A2 | A3 | A4 | A6 | A7 | L101 L73 L89 L52 L50 L48 | A13 | A15 | A17 | L99 L88 L91 L92 L86 L84 L78 | A19 | L113 L116 L117 L118 L128 L120 L121 L122 L129 L126 L125 L124 L114 L115 | L151 L150 L154 L152 L153 L149 L148 L147 | L157 L156 L155 | L158 L159 A22 A23 L160 | L161 L165 A21 L166 | L162 L163 A20 L164 | A25 | L197 A27 L196 L209 L242 L219 L218 L216 L194 L193 L188 | L210 L242 L244 L240 L221 L239 L243 L241 L223 L213 | L208 L190 L189 L253 L226 L229 A35 L227 L249 L254 L255 L341 L344 L256 L343 L342 L350 L351 L247 L248 L230 L303 L302 A41 L305 L298 L300 A31 L308 L206 L205 A30 L207 L204 L200 L202 L290 L289 L288 L283 L284 L282 L286 L287 L203 L330 A51 L328 L320 L334 L335 A47 L321 L294 L296 A44 L318 L316 L214 L215 L242 L223 L241 L243 L239 L221 L240 L244 | L251 L254 L247 L351 L350 L342 L343 L256 L344 L341 L255 | L290 L287 L286 L282 L284 L283 L288 L289 L281 | L233 L234 L232 L231 L225 L252 L191 | L193 L195 L212 A33 L211 L317 L272 L313 | A26 | L198 L332 L333 L327 A49 L331 L319 L329 A50 L201 L199 | A28 | A29 | A32 | L222 L224 L245 L276 L277 L246 L238 L220 | A34 | L236 L237 L235 | L257 L262 L348 L266 L346 L347 L345 L267 L258 L265 L264 L263 L261 L260 L259 | L268 A36 L278 L274 | L280 L270 A37 L269 | L279 L275 A38 A39 L271 | L273 L295 L323 A48 L322 L324 L293 | L292 L315 L311 L309 L337 L326 | L306 L304 L307 L301 L299 L297 | A40 | A42 | A43 | A45 | A46 | L338 L339 L340 bodies 4
sketch "Sketch14" plane through (0, 0, 0) normal (0, 0, -1) x (-1, 0, 0)
  line L0 (-63.5, 75.0796) -> (-63.5, 88.9) projected
  line L1 (0, 0) -> (-63.5, 0)
  line L2 (-63.5, 0) -> (-63.5, 88.9)
  line L3 (-63.5, 88.9) -> (0, 88.9)
  line L4 (0, 88.9) -> (0, 0)
  line L5 (-62.5, 1) -> (-1, 1)
  line L6 (-1, 1) -> (-1, 87.9)
  line L7 (-1, 87.9) -> (-62.5, 87.9)
  line L8 (-62.5, 87.9) -> (-62.5, 1)
  dimension "d90" = 1
  constraints: 16 end point, 4 parallel, 2 perpendicular, 1 horizontal, 3 other
  measures "d90" distance between parallel lines of L1 L5
extrude "Extrusion18" add sketch "Sketch14" along normal blind 0.2 separate body contours L8 L7 L6 L5
sketch "Sketch16" plane through (0, 0, 0) normal (0, 0, -1) x (-1, 0, 0)
  line L0 (-1, 1) -> (-1, 87.9) projected
  line L1 (-1, 87.9) -> (-62.5, 87.9) projected
  line L2 (-62.5, 87.9) -> (-62.5, 1) projected
  line L3 (-62.5, 1) -> (-1, 1) projected
  line L4 (0, 88.9) -> (0, 75.0796) projected
  line L5 (-31.75, 0) -> (-63.5, 0) projected
  line L6 (0, 88.9) -> (-63.5, 88.9)
  line L7 (-63.5, 88.9) -> (-63.5, 0)
  line L8 (-63.5, 0) -> (0, 0)
  line L9 (0, 0) -> (0, 88.9)
  constraints: 8 end point, 2 parallel, 1 horizontal, 1 perpendicular
extrude "Extrusion19" add sketch "Sketch16" along normal blind 0.2 bodies 3
sketch "Sketch17" plane through (0, 0, -0.2) normal (0, 0, -1) x (-1, 0, 0)
  line L0 (-63.5, 88.9) -> (-63.5, 0)
  line L1 (-63.5, 0) -> (0, 0)
  line L2 (0, 0) -> (0, 88.9)
  line L3 (0, 88.9) -> (-63.5, 88.9)
  line L4 (-62.5, 1) -> (-62.5, 87.9) construction
  line L5 (-62.5, 44.45) -> (-1, 44.45) construction
  line L6 (-1, 87.9) -> (-1, 1) construction
  line L7 (-57.9556, 87.392) -> (-49.5403, 87.392) construction
  line L8 (-49.5403, 87.392) -> (-49.5403, 73.7102) construction
  line L9 (-49.5403, 73.7102) -> (-57.9556, 73.7102) construction
  line L10 (-57.9556, 73.7102) -> (-57.9556, 87.392) construction
  line L11 (-5.5444, 1.508) -> (-13.9597, 1.508) construction
  line L12 (-13.9597, 1.508) -> (-13.9597, 15.8789) construction
  line L13 (-13.9597, 15.8789) -> (-5.5444, 15.8789) construction
  line L14 (-5.5444, 15.8789) -> (-5.5444, 1.508) construction
  line L15 (-62.5, 87.9) -> (-1, 87.9) projected
  line L16 (-1, 1) -> (-62.5, 1) projected
  arc A0 (-30.2318, 152.8359) -> (-29.2741, 152.992) centre (-30.7695, 159.15) ccw
  arc A1 (-29.2741, 152.992) -> (-28.3624, 153.2915) centre (-30.7051, 158.8848) ccw
  arc A2 (-28.3624, 153.2915) -> (-27.5102, 153.7308) centre (-30.7007, 158.8742) ccw
  arc A3 (-27.5102, 153.7308) -> (-26.7295, 154.3028) centre (-30.8216, 159.0691) ccw
  arc A4 (-26.7295, 154.3028) -> (-26.5602, 154.4555) centre (-29.7762, 157.8515) ccw
  arc A5 (-26.5602, 154.4555) -> (-26.3661, 154.6447) centre (-32.9458, 161.1985) ccw
  arc A6 (-26.3661, 154.6447) -> (-26.1868, 154.8299) centre (-32.7882, 161.0414) ccw
  arc A7 (-26.1868, 154.8299) -> (-26.0716, 154.9633) centre (-27.6947, 156.2487) ccw
  line L17 (-26.0716, 154.9633) -> (-26.0141, 155.0359)
  line L18 (-26.0141, 155.0359) -> (-26.3954, 155.3869)
  line L19 (-26.3954, 155.3869) -> (-26.7767, 155.7379)
  line L20 (-26.7767, 155.7379) -> (-26.8787, 155.6215)
  arc A8 (-27.4766, 155.0393) -> (-26.8787, 155.6215) centre (-30.8226, 159.074) ccw
  arc A9 (-28.1597, 154.5591) -> (-27.4766, 155.0393) centre (-30.8288, 159.0814) ccw
  arc A10 (-28.9036, 154.1971) -> (-28.1597, 154.5591) centre (-30.7794, 158.9977) ccw
  arc A11 (-29.6826, 153.9666) -> (-28.9036, 154.1971) centre (-30.6484, 158.6625) ccw
  arc A12 (-30.1963, 153.8885) -> (-29.6826, 153.9666) centre (-30.6931, 158.8802) ccw
  arc A13 (-30.7227, 153.8623) -> (-30.1963, 153.8885) centre (-30.7227, 159.1776) ccw
  arc A14 (-31.2492, 153.8885) -> (-30.7227, 153.8623) centre (-30.7227, 159.1776) ccw
  arc A15 (-31.7628, 153.9666) -> (-31.2492, 153.8885) centre (-30.7523, 158.8802) ccw
  arc A16 (-32.5419, 154.1968) -> (-31.7628, 153.9666) centre (-30.7929, 158.6827) ccw
  arc A17 (-33.2838, 154.5574) -> (-32.5419, 154.1968) centre (-30.6831, 158.9644) ccw
  arc A18 (-33.9658, 155.0371) -> (-33.2838, 154.5574) centre (-30.626, 159.0611) ccw
  arc A19 (-34.5666, 155.6213) -> (-33.9658, 155.0371) centre (-30.5582, 159.1428) ccw
  line L21 (-34.5666, 155.6213) -> (-34.6687, 155.7375)
  line L22 (-34.6687, 155.7375) -> (-35.0502, 155.3869)
  line L23 (-35.0502, 155.3869) -> (-35.4317, 155.0364)
  line L24 (-35.4317, 155.0364) -> (-35.3718, 154.9592)
  arc A20 (-35.3718, 154.9592) -> (-35.247, 154.8167) centre (-34.1122, 155.9365) ccw
  arc A21 (-35.247, 154.8167) -> (-34.9997, 154.5715) centre (-24.0403, 165.8759) ccw
  arc A22 (-34.9997, 154.5715) -> (-34.7417, 154.3276) centre (-25.0154, 164.8702) ccw
  arc A23 (-34.7417, 154.3276) -> (-34.5555, 154.1677) centre (-32.4264, 156.8372) ccw
  arc A24 (-34.5555, 154.1677) -> (-33.7925, 153.6456) centre (-30.6112, 159.1131) ccw
  arc A25 (-33.7925, 153.6456) -> (-32.9694, 153.2465) centre (-30.7414, 158.8893) ccw
  arc A26 (-32.9694, 153.2465) -> (-32.0946, 152.9752) centre (-30.7362, 158.9026) ccw
  arc A27 (-32.0946, 152.9752) -> (-31.1778, 152.8341) centre (-30.666, 159.2088) ccw
  arc A28 (-31.1778, 152.8341) -> (-30.9548, 152.8216) centre (-30.8064, 157.4603) ccw
  arc A29 (-30.9548, 152.8216) -> (-30.7033, 152.8178) centre (-30.7168, 160.2595) ccw
  arc A30 (-30.7033, 152.8178) -> (-30.4526, 152.8225) centre (-30.7168, 160.2266) ccw
  arc A31 (-30.4526, 152.8225) -> (-30.2318, 152.8359) centre (-30.6126, 157.3075) ccw
  arc A32 (-30.2318, 154.5347) -> (-29.6439, 154.6443) centre (-30.8055, 159.2456) ccw
  arc A33 (-29.6439, 154.6443) -> (-29.0861, 154.8255) centre (-30.7184, 158.9003) ccw
  arc A34 (-29.0861, 154.8255) -> (-28.5561, 155.08) centre (-30.7266, 158.9209) ccw
  arc A35 (-28.5561, 155.08) -> (-28.0512, 155.4082) centre (-30.9453, 159.3079) ccw
  arc A36 (-28.0512, 155.4082) -> (-27.8884, 155.5423) centre (-29.2999, 157.0908) ccw
  arc A37 (-27.8884, 155.5423) -> (-27.6412, 155.7736) centre (-36.5633, 165.0596) ccw
  arc A38 (-27.6412, 155.7736) -> (-27.4009, 156.0096) centre (-38.3112, 166.8788) ccw
  arc A39 (-27.4009, 156.0096) -> (-27.3015, 156.1285) centre (-28.03, 156.6362) ccw
  line L25 (-27.3015, 156.1285) -> (-27.2617, 156.1856)
  line L26 (-27.2617, 156.1856) -> (-27.6402, 156.5429)
  line L27 (-27.6402, 156.5429) -> (-28.0186, 156.9002)
  line L28 (-28.0186, 156.9002) -> (-28.096, 156.8068)
  arc A40 (-28.4105, 156.4711) -> (-28.096, 156.8068) centre (-30.9967, 159.2091) ccw
  arc A41 (-28.7563, 156.185) -> (-28.4105, 156.4711) centre (-30.7534, 158.9515) ccw
  arc A42 (-29.1314, 155.9507) -> (-28.7563, 156.185) centre (-30.6939, 158.8691) ccw
  arc A43 (-29.5333, 155.7693) -> (-29.1314, 155.9507) centre (-30.6751, 158.834) ccw
  arc A44 (-30.5648, 155.5565) -> (-29.5333, 155.7693) centre (-30.7378, 159.0023) ccw
  arc A45 (-31.6014, 155.6685) -> (-30.5648, 155.5565) centre (-30.7312, 158.8698) ccw
  arc A46 (-32.5561, 156.0977) -> (-31.6014, 155.6685) centre (-30.7238, 158.8971) ccw
  arc A47 (-33.3493, 156.8066) -> (-32.5561, 156.0977) centre (-30.604, 159.08) ccw
  line L29 (-33.3493, 156.8066) -> (-33.4265, 156.8998)
  line L30 (-33.4265, 156.8998) -> (-33.8047, 156.5423)
  line L31 (-33.8047, 156.5423) -> (-34.1829, 156.1847)
  line L32 (-34.1829, 156.1847) -> (-34.1433, 156.1281)
  arc A48 (-34.1433, 156.1281) -> (-34.1157, 156.0937) centre (-33.873, 156.3168) ccw
  arc A49 (-34.1157, 156.0937) -> (-34.0403, 156.0126) centre (-27.3184, 162.3393) ccw
  arc A50 (-34.0403, 156.0126) -> (-33.949, 155.9171) centre (-27.8592, 161.8304) ccw
  arc A51 (-33.949, 155.9171) -> (-33.8482, 155.8145) centre (-25.4382, 164.1812) ccw
  arc A52 (-33.8482, 155.8145) -> (-33.5622, 155.5485) centre (-30.2631, 159.3811) ccw
  arc A53 (-33.5622, 155.5485) -> (-33.2726, 155.3216) centre (-30.9641, 158.5667) ccw
  arc A54 (-33.2726, 155.3216) -> (-32.9638, 155.1228) centre (-30.9724, 158.555) ccw
  arc A55 (-32.9638, 155.1228) -> (-32.6202, 154.941) centre (-30.4654, 159.429) ccw
  arc A56 (-32.6202, 154.941) -> (-32.2788, 154.7952) centre (-30.8009, 158.7303) ccw
  arc A57 (-32.2788, 154.7952) -> (-31.9189, 154.6769) centre (-30.6765, 159.0613) ccw
  arc A58 (-31.9189, 154.6769) -> (-31.5499, 154.5887) centre (-30.6733, 159.0727) ccw
  arc A59 (-31.5499, 154.5887) -> (-31.1813, 154.5333) centre (-30.7325, 158.7697) ccw
  arc A60 (-31.1813, 154.5333) -> (-30.984, 154.5203) centre (-30.9195, 157.0051) ccw
  arc A61 (-30.984, 154.5203) -> (-30.6981, 154.5168) centre (-30.7139, 164.9247) ccw
  arc A62 (-30.6981, 154.5168) -> (-30.4147, 154.521) centre (-30.7142, 165.0774) ccw
  arc A63 (-30.4147, 154.521) -> (-30.2318, 154.5347) centre (-30.4708, 156.4969) ccw
  arc A64 (-30.5339, 156.2056) -> (-30.0457, 156.2906) centre (-30.8617, 159.5345) ccw
  arc A65 (-30.0457, 156.2906) -> (-29.6028, 156.4442) centre (-30.7001, 158.8922) ccw
  arc A66 (-29.6028, 156.4442) -> (-29.2021, 156.6688) centre (-30.6528, 158.7867) ccw
  arc A67 (-29.2021, 156.6688) -> (-28.8398, 156.965) centre (-30.7651, 158.9506) ccw
  arc A68 (-28.8398, 156.965) -> (-28.7235, 157.0826) centre (-31.6576, 159.8709) ccw
  arc A69 (-28.7235, 157.0826) -> (-28.6125, 157.2042) centre (-31.6085, 159.8243) ccw
  arc A70 (-28.6125, 157.2042) -> (-28.5158, 157.317) centre (-34.328, 162.2026) ccw
  arc A71 (-28.5158, 157.317) -> (-28.5043, 157.3487) centre (-28.5535, 157.3487) ccw
  arc A72 (-28.5043, 157.3487) -> (-28.5102, 157.3623) centre (-28.523, 157.3487) ccw
  arc A73 (-28.5102, 157.3623) -> (-28.8745, 157.7054) centre (-931.3716, -801.1568) ccw
  arc A74 (-28.8745, 157.7054) -> (-29.234, 158.0435) centre (-490.9775, -333.258) ccw
  arc A75 (-29.234, 158.0435) -> (-29.2594, 158.0595) centre (-29.2874, 157.9867) ccw
  arc A76 (-29.2594, 158.0595) -> (-29.2682, 158.0575) centre (-29.2623, 158.0519) ccw
  arc A77 (-29.2682, 158.0575) -> (-29.2946, 158.0285) centre (-28.4914, 157.323) ccw
  arc A78 (-29.2946, 158.0285) -> (-29.3253, 157.9913) centre (-28.7021, 157.508) ccw
  arc A79 (-29.3253, 157.9913) -> (-29.3589, 157.9462) centre (-28.1664, 157.0926) ccw
  arc A80 (-29.5609, 157.7139) -> (-29.3589, 157.9462) centre (-30.6858, 158.8959) ccw
  arc A81 (-29.8051, 157.5206) -> (-29.5609, 157.7139) centre (-30.7411, 158.9541) ccw
  arc A82 (-30.0819, 157.3737) -> (-29.8051, 157.5206) centre (-30.7523, 158.9712) ccw
  arc A83 (-30.3802, 157.2793) -> (-30.0819, 157.3737) centre (-30.7491, 158.9635) ccw
  arc A84 (-30.5552, 157.2562) -> (-30.3802, 157.2793) centre (-30.6043, 158.3025) ccw
  arc A85 (-30.7819, 157.2547) -> (-30.5552, 157.2562) centre (-30.6864, 160.051) ccw
  arc A86 (-31.0081, 157.2717) -> (-30.7819, 157.2547) centre (-30.6863, 160.0531) ccw
  arc A87 (-31.1819, 157.3067) -> (-31.0081, 157.2717) centre (-30.8861, 158.3262) ccw
  arc A88 (-31.4472, 157.4107) -> (-31.1819, 157.3067) centre (-30.7468, 158.8063) ccw
  arc A89 (-31.7021, 157.5652) -> (-31.4472, 157.4107) centre (-30.6085, 159.082) ccw
  arc A90 (-31.9285, 157.7577) -> (-31.7021, 157.5652) centre (-30.6158, 159.0719) ccw
  arc A91 (-32.1084, 157.9747) -> (-31.9285, 157.7577) centre (-30.8627, 158.8246) ccw
  arc A92 (-32.1084, 157.9747) -> (-32.1332, 158.0091) centre (-32.7619, 157.5288) ccw
  arc A93 (-32.1332, 158.0091) -> (-32.1566, 158.0371) centre (-32.4793, 157.7447) ccw
  arc A94 (-32.1566, 158.0371) -> (-32.1767, 158.0579) centre (-32.485, 157.7395) ccw
  arc A95 (-32.1767, 158.0579) -> (-32.1854, 158.0597) centre (-32.1824, 158.0519) ccw
  arc A96 (-32.1854, 158.0597) -> (-32.21, 158.0443) centre (-32.1586, 157.9895) ccw
  arc A97 (-32.21, 158.0443) -> (-32.5704, 157.7059) centre (465.2262, -372.1602) ccw
  arc A98 (-32.5704, 157.7059) -> (-32.9355, 157.3628) centre (930.9989, -867.9399) ccw
  arc A99 (-32.9355, 157.3628) -> (-32.9412, 157.3496) centre (-32.9231, 157.3496) ccw
  arc A100 (-32.9412, 157.3496) -> (-32.9394, 157.3442) centre (-32.9321, 157.3496) ccw
  arc A101 (-32.9394, 157.3442) -> (-32.9135, 157.3094) centre (-26.8123, 161.8634) ccw
  arc A102 (-32.9135, 157.3094) -> (-32.8832, 157.2695) centre (-30.7865, 158.897) ccw
  arc A103 (-32.8832, 157.2695) -> (-32.8471, 157.2236) centre (-29.0549, 160.2412) ccw
  arc A104 (-32.8471, 157.2236) -> (-32.6598, 157.0163) centre (-31.1019, 158.6123) ccw
  arc A105 (-32.6598, 157.0163) -> (-32.4283, 156.8103) centre (-30.309, 159.4247) ccw
  arc A106 (-32.4283, 156.8103) -> (-32.1782, 156.6259) centre (-30.2991, 159.4368) ccw
  arc A107 (-32.1782, 156.6259) -> (-31.9345, 156.4838) centre (-30.9004, 158.5374) ccw
  arc A108 (-31.9345, 156.4838) -> (-31.7777, 156.4145) centre (-31.1715, 157.999) ccw
  arc A109 (-31.7777, 156.4145) -> (-31.5739, 156.3425) centre (-30.263, 160.3734) ccw
  arc A110 (-31.5739, 156.3425) -> (-31.3657, 156.2806) centre (-30.2572, 160.3914) ccw
  arc A111 (-31.3657, 156.2806) -> (-31.1947, 156.2432) centre (-30.8941, 158.0293) ccw
  arc A112 (-31.1947, 156.2432) -> (-31.0412, 156.2232) centre (-30.8445, 158.3243) ccw
  arc A113 (-31.0412, 156.2232) -> (-30.8453, 156.2084) centre (-30.539, 161.5866) ccw
  arc A114 (-30.8453, 156.2084) -> (-30.6563, 156.2009) centre (-30.5362, 161.6352) ccw
  arc A115 (-30.6563, 156.2009) -> (-30.5339, 156.2056) centre (-30.6338, 157.2199) ccw
  arc A116 (-30.5056, 157.9205) -> (-30.2505, 158.0387) centre (-30.7396, 158.76) ccw
  arc A117 (-30.2505, 158.0387) -> (-30.0441, 158.2327) centre (-30.7538, 158.781) ccw
  arc A118 (-30.0441, 158.2327) -> (-29.9099, 158.4796) centre (-30.7418, 158.7717) ccw
  arc A119 (-29.9099, 158.4796) -> (-29.8639, 158.7512) centre (-30.6789, 158.7496) ccw
  arc A120 (-29.8639, 158.7512) -> (-29.9519, 159.1258) centre (-30.7118, 158.7495) ccw
  arc A121 (-29.9519, 159.1258) -> (-30.1969, 159.4268) centre (-30.737, 158.737) ccw
  arc A122 (-30.1969, 159.4268) -> (-30.5464, 159.5911) centre (-30.7307, 158.7451) ccw
  arc A123 (-30.5464, 159.5911) -> (-30.9268, 159.5834) centre (-30.7205, 158.7916) ccw
  arc A124 (-30.9268, 159.5834) -> (-31.1466, 159.4956) centre (-30.688, 158.6667) ccw
  arc A125 (-31.1466, 159.4956) -> (-31.3287, 159.3584) centre (-30.7512, 158.781) ccw
  arc A126 (-31.3287, 159.3584) -> (-31.4658, 159.1763) centre (-30.7513, 158.781) ccw
  arc A127 (-31.4658, 159.1763) -> (-31.5536, 158.9565) centre (-30.6369, 158.7177) ccw
  arc A128 (-31.5536, 158.9565) -> (-31.5609, 158.5719) centre (-30.7575, 158.7492) ccw
  arc A129 (-31.5609, 158.5719) -> (-31.3931, 158.2209) centre (-30.7233, 158.7567) ccw
  arc A130 (-31.3931, 158.2209) -> (-31.086, 157.978) centre (-30.713, 158.765) ccw
  arc A131 (-31.086, 157.978) -> (-30.7046, 157.8951) centre (-30.7173, 158.7558) ccw
  arc A132 (-30.7046, 157.8951) -> (-30.6547, 157.8975) centre (-30.7159, 158.6587) ccw
  arc A133 (-30.6547, 157.8975) -> (-30.5991, 157.9033) centre (-30.7509, 159.0939) ccw
  arc A134 (-30.5991, 157.9033) -> (-30.5463, 157.9113) centre (-30.7426, 159.0287) ccw
  arc A135 (-30.5463, 157.9113) -> (-30.5056, 157.9205) centre (-30.62, 158.3308) ccw
  arc A136 (-33.4163, 54.0207) -> (-36.541, 53.5113) centre (-31.6621, 33.4199) ccw
  arc A137 (-36.541, 53.5113) -> (-39.5155, 52.5341) centre (-31.8722, 34.2851) ccw
  arc A138 (-39.5155, 52.5341) -> (-42.2961, 51.1009) centre (-31.8866, 34.3196) ccw
  arc A139 (-42.2961, 51.1009) -> (-44.8431, 49.2347) centre (-31.4921, 33.6837) ccw
  arc A140 (-44.8431, 49.2347) -> (-45.3957, 48.7364) centre (-34.9028, 37.6564) ccw
  arc A141 (-45.3957, 48.7364) -> (-46.0288, 48.119) centre (-24.5615, 26.7364) ccw
  arc A142 (-46.0288, 48.119) -> (-46.6138, 47.5148) centre (-25.0759, 27.2488) ccw
  arc A143 (-46.6138, 47.5148) -> (-46.9896, 47.0797) centre (-41.6942, 42.8857) ccw
  line L33 (-46.9896, 47.0797) -> (-47.1772, 46.8428)
  line L34 (-47.1772, 46.8428) -> (-45.9332, 45.6975)
  line L35 (-45.9332, 45.6975) -> (-44.6891, 44.5522)
  line L36 (-44.6891, 44.5522) -> (-44.3566, 44.9321)
  arc A144 (-42.4056, 46.8317) -> (-44.3566, 44.9321) centre (-31.489, 33.6679) ccw
  arc A145 (-40.1769, 48.3985) -> (-42.4056, 46.8317) centre (-31.4688, 33.6437) ccw
  arc A146 (-37.7497, 49.5795) -> (-40.1769, 48.3985) centre (-31.6299, 33.9167) ccw
  arc A147 (-35.2082, 50.3314) -> (-37.7497, 49.5795) centre (-32.0573, 35.0104) ccw
  arc A148 (-33.5324, 50.5864) -> (-35.2082, 50.3314) centre (-31.9113, 34.3003) ccw
  arc A149 (-31.8147, 50.6717) -> (-33.5324, 50.5864) centre (-31.8147, 33.3299) ccw
  arc A150 (-30.097, 50.5864) -> (-31.8147, 50.6717) centre (-31.8147, 33.3299) ccw
  arc A151 (-28.4213, 50.3314) -> (-30.097, 50.5864) centre (-31.7182, 34.3003) ccw
  arc A152 (-25.8794, 49.5804) -> (-28.4213, 50.3314) centre (-31.5857, 34.9446) ccw
  arc A153 (-23.4588, 48.4038) -> (-25.8794, 49.5804) centre (-31.944, 34.0255) ccw
  arc A154 (-21.2337, 46.8388) -> (-23.4588, 48.4038) centre (-32.1303, 33.7098) ccw
  arc A155 (-19.2735, 44.9329) -> (-21.2337, 46.8388) centre (-32.3516, 33.4432) ccw
  line L37 (-19.2735, 44.9329) -> (-18.9403, 44.5537)
  line L38 (-18.9403, 44.5537) -> (-17.6957, 45.6975)
  line L39 (-17.6957, 45.6975) -> (-16.451, 46.8412)
  line L40 (-16.451, 46.8412) -> (-16.6464, 47.093)
  arc A156 (-16.6464, 47.093) -> (-17.0536, 47.558) centre (-20.7559, 43.9044) ccw
  arc A157 (-17.0536, 47.558) -> (-17.8605, 48.3578) centre (-53.6172, 11.4756) ccw
  arc A158 (-17.8605, 48.3578) -> (-18.7022, 49.1538) centre (-50.4359, 14.7571) ccw
  arc A159 (-18.7022, 49.1538) -> (-19.3099, 49.6753) centre (-26.2562, 40.9659) ccw
  arc A160 (-19.3099, 49.6753) -> (-21.7992, 51.3787) centre (-32.1786, 33.5403) ccw
  arc A161 (-21.7992, 51.3787) -> (-24.4848, 52.681) centre (-31.7538, 34.2705) ccw
  arc A162 (-24.4848, 52.681) -> (-27.3389, 53.566) centre (-31.7709, 34.2271) ccw
  arc A163 (-27.3389, 53.566) -> (-30.3299, 54.0263) centre (-31.9998, 33.2282) ccw
  arc A164 (-30.3299, 54.0263) -> (-31.0576, 54.0671) centre (-31.5418, 38.9328) ccw
  arc A165 (-31.0576, 54.0671) -> (-31.8781, 54.0795) centre (-31.834, 29.8) ccw
  arc A166 (-31.8781, 54.0795) -> (-32.6962, 54.0642) centre (-31.8342, 29.9074) ccw
  arc A167 (-32.6962, 54.0642) -> (-33.4163, 54.0207) centre (-32.174, 39.4315) ccw
  arc A168 (-33.4163, 48.478) -> (-35.3347, 48.1205) centre (-31.5446, 33.1082) ccw
  arc A169 (-35.3347, 48.1205) -> (-37.1546, 47.5292) centre (-31.829, 34.2345) ccw
  arc A170 (-37.1546, 47.5292) -> (-38.8837, 46.6988) centre (-31.8021, 34.1673) ccw
  arc A171 (-38.8837, 46.6988) -> (-40.5311, 45.6279) centre (-31.0886, 32.9048) ccw
  arc A172 (-40.5311, 45.6279) -> (-41.0622, 45.1907) centre (-36.4569, 40.1382) ccw
  arc A173 (-41.0622, 45.1907) -> (-41.8688, 44.4358) centre (-12.7592, 14.1391) ccw
  arc A174 (-41.8688, 44.4358) -> (-42.6526, 43.6661) centre (-7.0561, 8.2035) ccw